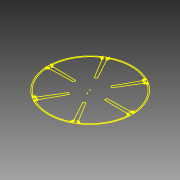
# Autodesk Inventor part: Wheel-190D-Join
Saved by Autodesk Inventor 2014 SP1 (Build 180222100, 222)
## iProperties
Created: 2017-01-25
Part Number: Wheel-190D-Join
Material: Generic
Document SubType Name: Modeling
Designer: danielsikar
Density: 1 g/cm^3
Appearance: Default
Author: danielsikar
Autodesk Inventor part; units mm, degrees
ref_plane "YZ Plane" through (0, 0, 0) normal (1, 0, 0) x (0, 1, 0)
ref_plane "XZ Plane" through (0, 0, 0) normal (0, 1, 0) x (-1, 0, 0)
ref_plane "XY Plane" through (0, 0, 0) normal (0, 0, 1) x (1, 0, 0)
sketch "Sketch1" plane through (0, 0, 0) normal (0, 0, 1) x (1, 0, 0)
  arc A0 (31.6369, 7.0811) -> (31.6369, 12.2394) centre (-3.2679, 9.6603) ccw
  line L0 (31.6369, 12.2394) -> (85.6305, 13.4951)
  spline S0 degree 3 poles (88.553, 15.6009) (88.5581, 15.5214) (88.5526, 15.4427) (88.5217, 15.2843) (88.4962, 15.2066) (88.3926, 14.9703) (88.2868, 14.8191) (87.9731, 14.4565) (87.7042, 14.2313) (87.1267, 13.8761) (86.8348, 13.7414) (86.2409, 13.5562) (85.9366, 13.5022) (85.6305, 13.4951) knots 0 0 0 0 0.068577 0.068577 0.138951 0.138951 0.290932 0.290932 0.552904 0.552904 0.779743 0.779743 1 1 1 1
  arc A1 (88.553, 15.6009) -> (47.7872, 86.2092) centre (-3.2679, 9.6603) ccw
  spline S1 degree 3 poles (44.5024, 84.7311) (44.7113, 85.0744) (44.9886, 85.3747) (45.7206, 85.9508) (46.1829, 86.1728) (46.7972, 86.3435) (47.0239, 86.382) (47.3383, 86.3694) (47.4368, 86.3554) (47.6229, 86.3008) (47.7082, 86.2619) (47.7872, 86.2092) knots 0 0 0 0 0.278386 0.278386 0.644497 0.644497 0.831809 0.831809 0.917649 0.917649 1 1 1 1
  line L1 (16.4181, 38.5991) -> (44.5024, 84.7311)
  arc A2 (16.4181, 38.5991) -> (11.9508, 41.1783) centre (-3.2679, 9.6603) ccw
  line L2 (11.9508, 41.1783) -> (37.8602, 88.566)
  spline S2 degree 3 poles (37.4978, 92.1498) (37.6052, 92.0967) (37.6979, 92.0243) (37.8803, 91.8249) (37.9599, 91.6922) (38.1263, 91.328) (38.198, 91.0566) (38.2844, 90.4211) (38.2862, 90.026) (38.157, 89.2543) (38.0394, 88.8938) (37.8602, 88.566) knots 0 0 0 0 0.107871 0.107871 0.243625 0.243625 0.469812 0.469812 0.746518 0.746518 1 1 1 1
  arc A3 (37.4978, 92.1498) -> (-44.0337, 92.1498) centre (-3.2679, 9.6603) ccw
  spline S3 degree 3 poles (-44.3961, 88.566) (-44.5889, 88.9186) (-44.7103, 89.3089) (-44.8432, 90.2308) (-44.8043, 90.7422) (-44.645, 91.3596) (-44.565, 91.5752) (-44.3969, 91.8411) (-44.3355, 91.9195) (-44.1951, 92.0533) (-44.1189, 92.1077) (-44.0337, 92.1498) knots 0 0 0 0 0.278386 0.278386 0.644497 0.644497 0.831809 0.831809 0.917649 0.917649 1 1 1 1
  line L3 (-18.4867, 41.1783) -> (-44.3961, 88.566)
  arc A4 (-18.4867, 41.1783) -> (-22.954, 38.5991) centre (-3.2679, 9.6603) ccw
  line L4 (-22.954, 38.5991) -> (-51.0383, 84.7311)
  spline S4 degree 3 poles (-54.3231, 86.2092) (-54.2235, 86.2757) (-54.1144, 86.3197) (-53.8505, 86.3781) (-53.6958, 86.3806) (-53.2972, 86.3426) (-53.0263, 86.269) (-52.4327, 86.0261) (-52.0897, 85.8301) (-51.4859, 85.3323) (-51.2325, 85.0503) (-51.0383, 84.7311) knots 0 0 0 0 0.107871 0.107871 0.243625 0.243625 0.469812 0.469812 0.746518 0.746518 1 1 1 1
  arc A5 (-54.3231, 86.2092) -> (-95.0889, 15.6009) centre (-3.2679, 9.6603) ccw
  spline S5 degree 3 poles (-92.1664, 13.4951) (-92.5681, 13.5044) (-92.9668, 13.5944) (-93.8317, 13.9403) (-94.2552, 14.2297) (-94.7102, 14.6763) (-94.8569, 14.8534) (-95.0031, 15.132) (-95.0403, 15.2243) (-95.086, 15.4128) (-95.095, 15.5061) (-95.0889, 15.6009) knots 0 0 0 0 0.278386 0.278386 0.644497 0.644497 0.831809 0.831809 0.917649 0.917649 1 1 1 1
  line L5 (-38.1728, 12.2394) -> (-92.1664, 13.4951)
  arc A6 (-38.1728, 12.2394) -> (-38.1728, 7.0811) centre (-3.2679, 9.6603) ccw
  line L6 (-38.1728, 7.0811) -> (-92.1664, 5.8254)
  spline S6 degree 3 poles (-95.0889, 3.7196) (-95.0966, 3.8392) (-95.0802, 3.9557) (-94.9988, 4.2134) (-94.9236, 4.3486) (-94.6914, 4.6748) (-94.4922, 4.8726) (-93.9851, 5.2652) (-93.6438, 5.4643) (-92.9108, 5.7383) (-92.5399, 5.8167) (-92.1664, 5.8254) knots 0 0 0 0 0.107871 0.107871 0.243625 0.243625 0.469812 0.469812 0.746518 0.746518 1 1 1 1
  arc A7 (-95.0889, 3.7196) -> (-54.3231, -66.8887) centre (-3.2679, 9.6603) ccw
  spline S7 degree 3 poles (-51.0383, -65.4106) (-51.2472, -65.7539) (-51.5245, -66.0542) (-52.2565, -66.6303) (-52.7188, -66.8523) (-53.3331, -67.023) (-53.5598, -67.0615) (-53.8742, -67.0489) (-53.9727, -67.0349) (-54.1588, -66.9803) (-54.2441, -66.9414) (-54.3231, -66.8887) knots 0 0 0 0 0.278386 0.278386 0.644497 0.644497 0.831809 0.831809 0.917649 0.917649 1 1 1 1
  line L7 (-22.954, -19.2786) -> (-51.0383, -65.4106)
  arc A8 (-22.954, -19.2786) -> (-18.4867, -21.8578) centre (-3.2679, 9.6603) ccw
  line L8 (-18.4867, -21.8578) -> (-44.3961, -69.2455)
  spline S8 degree 3 poles (-44.0337, -72.8293) (-44.1411, -72.7762) (-44.2338, -72.7038) (-44.4162, -72.5044) (-44.4958, -72.3717) (-44.6622, -72.0075) (-44.7339, -71.7361) (-44.8203, -71.1006) (-44.8221, -70.7055) (-44.6929, -69.9338) (-44.5753, -69.5733) (-44.3961, -69.2455) knots 0 0 0 0 0.107871 0.107871 0.243625 0.243625 0.469812 0.469812 0.746518 0.746518 1 1 1 1
  arc A9 (-44.0337, -72.8293) -> (37.4978, -72.8293) centre (-3.2679, 9.6603) ccw
  spline S9 degree 3 poles (37.8602, -69.2455) (38.053, -69.598) (38.1744, -69.9884) (38.3073, -70.9103) (38.2684, -71.4217) (38.1091, -72.0391) (38.0291, -72.2547) (37.861, -72.5206) (37.7996, -72.599) (37.6592, -72.7328) (37.583, -72.7872) (37.4978, -72.8293) knots 0 0 0 0 0.278386 0.278386 0.644497 0.644497 0.831809 0.831809 0.917649 0.917649 1 1 1 1
  line L9 (11.9508, -21.8578) -> (37.8602, -69.2455)
  arc A10 (11.9508, -21.8578) -> (16.4181, -19.2786) centre (-3.2679, 9.6603) ccw
  line L10 (16.4181, -19.2786) -> (44.5024, -65.4106)
  spline S10 degree 3 poles (47.7872, -66.8887) (47.6876, -66.9552) (47.5785, -66.9992) (47.3146, -67.0575) (47.1599, -67.0601) (46.7613, -67.0221) (46.4904, -66.9484) (45.8968, -66.7056) (45.5538, -66.5096) (44.95, -66.0118) (44.6966, -65.7298) (44.5024, -65.4106) knots 0 0 0 0 0.107871 0.107871 0.243625 0.243625 0.469812 0.469812 0.746518 0.746518 1 1 1 1
  arc A11 (47.7872, -66.8887) -> (88.553, 3.7196) centre (-3.2679, 9.6603) ccw
  spline S11 degree 3 poles (85.6305, 5.8254) (86.0322, 5.8161) (86.4309, 5.7261) (87.2958, 5.3802) (87.7193, 5.0908) (88.1743, 4.6442) (88.321, 4.4671) (88.4672, 4.1885) (88.5044, 4.0962) (88.5501, 3.9077) (88.5591, 3.8144) (88.553, 3.7196) knots 0 0 0 0 0.278386 0.278386 0.644497 0.644497 0.831809 0.831809 0.917649 0.917649 1 1 1 1
  line L11 (31.6369, 7.0811) -> (85.6305, 5.8254)
  line L12 (90.9918, 13.6198) -> (91.074, 10.0868)
  arc A12 (47.291, -69.9913) -> (91.074, 10.0868) centre (-3.2679, 9.6603) ccw
  line L13 (47.291, -69.9913) -> (40.5213, -74.1126)
  line L14 (40.4329, -73.9508) -> (40.5213, -74.1126)
  arc A13 (-46.9688, -73.9508) -> (40.4329, -73.9508) centre (-3.2679, 9.6603) ccw
  line L15 (-46.9688, -73.9508) -> (-53.9227, -70.1487)
  line L16 (-53.8269, -69.9913) -> (-53.9227, -70.1487)
  arc A14 (-97.5277, 5.7007) -> (-53.8269, -69.9913) centre (-3.2679, 9.6603) ccw
  line L17 (-97.5277, 5.7007) -> (-97.712, 13.6241)
  line L18 (-97.5277, 13.6198) -> (-97.712, 13.6241)
  arc A15 (-53.8269, 89.3118) -> (-97.5277, 13.6198) centre (-3.2679, 9.6603) ccw
  line L19 (-53.8269, 89.3118) -> (-47.0572, 93.4331)
  line L20 (-46.9688, 93.2714) -> (-47.0572, 93.4331)
  arc A16 (40.4329, 93.2714) -> (-46.9688, 93.2714) centre (-3.2679, 9.6603) ccw
  line L21 (40.4329, 93.2714) -> (47.3868, 89.4693)
  line L22 (47.291, 89.3118) -> (47.3868, 89.4693)
  arc A17 (90.9918, 13.6198) -> (47.291, 89.3118) centre (-3.2679, 9.6603) ccw
  point P0 (0, 0)
ref_plane "Work Plane1" through (6.7321, 7.6603, 6.5) normal (0, 0, -1) x (-1, 0, 0)
ref_plane "Work Plane2" through (-91.9966, 5.6978, 0) normal (0, 0, 1) x (1, 0, 0)
sketch "Sketch2" plane through (6.7321, 7.6603, 6.5) normal (0, 0, -1) x (-1, 0, 0)
  arc A0 (-24.9048, 4.5792) -> (-24.9048, -0.5792) centre (10, 2) ccw
  line L0 (-24.9048, 4.5792) -> (-78.8985, 5.8348)
  spline S0 degree 3 poles (-81.8209, 7.9406) (-81.8261, 7.8611) (-81.8206, 7.7825) (-81.7897, 7.6241) (-81.7641, 7.5464) (-81.6606, 7.31) (-81.5548, 7.1589) (-81.2411, 6.7962) (-80.9721, 6.571) (-80.3946, 6.2158) (-80.1028, 6.0812) (-79.5089, 5.8959) (-79.2045, 5.842) (-78.8985, 5.8348) knots 0 0 0 0 0.068577 0.068577 0.138951 0.138951 0.290932 0.290932 0.552904 0.552904 0.779743 0.779743 1 1 1 1
  arc A1 (-41.0552, 78.5489) -> (-81.8209, 7.9406) centre (10, 2) ccw
  spline S1 degree 3 poles (-37.7703, 77.0709) (-37.9792, 77.4141) (-38.2566, 77.7144) (-38.9885, 78.2905) (-39.4509, 78.5125) (-40.0652, 78.6833) (-40.2919, 78.7218) (-40.6062, 78.7092) (-40.7048, 78.6952) (-40.8909, 78.6405) (-40.9762, 78.6017) (-41.0552, 78.5489) knots 0 0 0 0 0.278386 0.278386 0.644497 0.644497 0.831809 0.831809 0.917649 0.917649 1 1 1 1
  line L1 (-9.6861, 30.9389) -> (-37.7703, 77.0709)
  arc A2 (-5.2188, 33.5181) -> (-9.6861, 30.9389) centre (10, 2) ccw
  line L2 (-5.2188, 33.5181) -> (-31.1282, 80.9057)
  spline S2 degree 3 poles (-30.7657, 84.4896) (-30.8731, 84.4365) (-30.9658, 84.364) (-31.1483, 84.1647) (-31.2278, 84.0319) (-31.3942, 83.6678) (-31.4659, 83.3963) (-31.5524, 82.7609) (-31.5541, 82.3658) (-31.4249, 81.594) (-31.3074, 81.2336) (-31.1282, 80.9057) knots 0 0 0 0 0.107871 0.107871 0.243625 0.243625 0.469812 0.469812 0.746518 0.746518 1 1 1 1
  arc A3 (50.7657, 84.4896) -> (-30.7657, 84.4896) centre (10, 2) ccw
  spline S3 degree 3 poles (51.1282, 80.9057) (51.3209, 81.2583) (51.4423, 81.6486) (51.5753, 82.5706) (51.5364, 83.082) (51.3771, 83.6993) (51.2971, 83.9149) (51.129, 84.1809) (51.0676, 84.2592) (50.9272, 84.393) (50.8509, 84.4475) (50.7657, 84.4896) knots 0 0 0 0 0.278386 0.278386 0.644497 0.644497 0.831809 0.831809 0.917649 0.917649 1 1 1 1
  line L3 (25.2188, 33.5181) -> (51.1282, 80.9057)
  arc A4 (29.6861, 30.9389) -> (25.2188, 33.5181) centre (10, 2) ccw
  line L4 (29.6861, 30.9389) -> (57.7703, 77.0709)
  spline S4 degree 3 poles (61.0552, 78.5489) (60.9555, 78.6154) (60.8464, 78.6595) (60.5826, 78.7178) (60.4278, 78.7203) (60.0293, 78.6823) (59.7583, 78.6087) (59.1648, 78.3659) (58.8217, 78.1698) (58.218, 77.672) (57.9646, 77.39) (57.7703, 77.0709) knots 0 0 0 0 0.107871 0.107871 0.243625 0.243625 0.469812 0.469812 0.746518 0.746518 1 1 1 1
  arc A5 (101.8209, 7.9406) -> (61.0552, 78.5489) centre (10, 2) ccw
  spline S5 degree 3 poles (98.8985, 5.8348) (99.3002, 5.8442) (99.6989, 5.9342) (100.5638, 6.28) (100.9872, 6.5694) (101.4422, 7.0161) (101.5889, 7.1931) (101.7352, 7.4717) (101.7724, 7.564) (101.8181, 7.7525) (101.8271, 7.8458) (101.8209, 7.9406) knots 0 0 0 0 0.278386 0.278386 0.644497 0.644497 0.831809 0.831809 0.917649 0.917649 1 1 1 1
  line L5 (44.9048, 4.5792) -> (98.8985, 5.8348)
  arc A6 (44.9048, -0.5792) -> (44.9048, 4.5792) centre (10, 2) ccw
  line L6 (44.9048, -0.5792) -> (98.8985, -1.8348)
  spline S6 degree 3 poles (101.8209, -3.9406) (101.8287, -3.8211) (101.8123, -3.7046) (101.7308, -3.4469) (101.6557, -3.3116) (101.4235, -2.9855) (101.2242, -2.7876) (100.7172, -2.395) (100.3759, -2.196) (99.6429, -1.922) (99.272, -1.8435) (98.8985, -1.8348) knots 0 0 0 0 0.107871 0.107871 0.243625 0.243625 0.469812 0.469812 0.746518 0.746518 1 1 1 1
  arc A7 (61.0552, -74.5489) -> (101.8209, -3.9406) centre (10, 2) ccw
  spline S7 degree 3 poles (57.7703, -73.0709) (57.9792, -73.4141) (58.2566, -73.7144) (58.9885, -74.2905) (59.4509, -74.5125) (60.0652, -74.6833) (60.2919, -74.7218) (60.6062, -74.7092) (60.7048, -74.6952) (60.8909, -74.6405) (60.9762, -74.6017) (61.0552, -74.5489) knots 0 0 0 0 0.278386 0.278386 0.644497 0.644497 0.831809 0.831809 0.917649 0.917649 1 1 1 1
  line L7 (29.6861, -26.9389) -> (57.7703, -73.0709)
  arc A8 (25.2188, -29.5181) -> (29.6861, -26.9389) centre (10, 2) ccw
  line L8 (25.2188, -29.5181) -> (51.1282, -76.9057)
  spline S8 degree 3 poles (50.7657, -80.4896) (50.8731, -80.4365) (50.9658, -80.364) (51.1483, -80.1647) (51.2278, -80.0319) (51.3942, -79.6678) (51.4659, -79.3963) (51.5524, -78.7609) (51.5541, -78.3658) (51.4249, -77.594) (51.3074, -77.2336) (51.1282, -76.9057) knots 0 0 0 0 0.107871 0.107871 0.243625 0.243625 0.469812 0.469812 0.746518 0.746518 1 1 1 1
  arc A9 (-30.7657, -80.4896) -> (50.7657, -80.4896) centre (10, 2) ccw
  spline S9 degree 3 poles (-31.1282, -76.9057) (-31.3209, -77.2583) (-31.4423, -77.6486) (-31.5753, -78.5706) (-31.5364, -79.082) (-31.3771, -79.6993) (-31.2971, -79.9149) (-31.129, -80.1809) (-31.0676, -80.2592) (-30.9272, -80.393) (-30.8509, -80.4475) (-30.7657, -80.4896) knots 0 0 0 0 0.278386 0.278386 0.644497 0.644497 0.831809 0.831809 0.917649 0.917649 1 1 1 1
  line L9 (-5.2188, -29.5181) -> (-31.1282, -76.9057)
  arc A10 (-9.6861, -26.9389) -> (-5.2188, -29.5181) centre (10, 2) ccw
  line L10 (-9.6861, -26.9389) -> (-37.7703, -73.0709)
  spline S10 degree 3 poles (-41.0552, -74.5489) (-40.9555, -74.6154) (-40.8464, -74.6595) (-40.5826, -74.7178) (-40.4278, -74.7203) (-40.0293, -74.6823) (-39.7583, -74.6087) (-39.1648, -74.3659) (-38.8217, -74.1698) (-38.218, -73.672) (-37.9646, -73.39) (-37.7703, -73.0709) knots 0 0 0 0 0.107871 0.107871 0.243625 0.243625 0.469812 0.469812 0.746518 0.746518 1 1 1 1
  arc A11 (-81.8209, -3.9406) -> (-41.0552, -74.5489) centre (10, 2) ccw
  spline S11 degree 3 poles (-78.8985, -1.8348) (-79.3002, -1.8442) (-79.6989, -1.9342) (-80.5638, -2.28) (-80.9872, -2.5694) (-81.4422, -3.0161) (-81.5889, -3.1931) (-81.7352, -3.4717) (-81.7724, -3.564) (-81.8181, -3.7525) (-81.8271, -3.8458) (-81.8209, -3.9406) knots 0 0 0 0 0.278386 0.278386 0.644497 0.644497 0.831809 0.831809 0.917649 0.917649 1 1 1 1
  line L11 (-24.9048, -0.5792) -> (-78.8985, -1.8348)
  line L12 (-84.2597, 5.9595) -> (-84.3419, 2.4266)
  arc A12 (-84.3419, 2.4266) -> (-40.5589, -77.6516) centre (10, 2) ccw
  line L13 (-40.5589, -77.6516) -> (-33.7892, -81.7728)
  line L14 (-33.7008, -81.6111) -> (-33.7892, -81.7728)
  arc A13 (-33.7008, -81.6111) -> (53.7008, -81.6111) centre (10, 2) ccw
  line L15 (53.7008, -81.6111) -> (60.6548, -77.809)
  line L16 (60.5589, -77.6516) -> (60.6548, -77.809)
  arc A14 (60.5589, -77.6516) -> (104.2597, -1.9595) centre (10, 2) ccw
  line L17 (104.2597, -1.9595) -> (104.444, 5.9638)
  line L18 (104.2597, 5.9595) -> (104.444, 5.9638)
  arc A15 (104.2597, 5.9595) -> (60.5589, 81.6516) centre (10, 2) ccw
  line L19 (60.5589, 81.6516) -> (53.7892, 85.7728)
  line L20 (53.7008, 85.6111) -> (53.7892, 85.7728)
  arc A16 (53.7008, 85.6111) -> (-33.7008, 85.6111) centre (10, 2) ccw
  line L21 (-33.7008, 85.6111) -> (-40.6548, 81.809)
  line L22 (-40.5589, 81.6516) -> (-40.6548, 81.809)
  arc A17 (-40.5589, 81.6516) -> (-84.2597, 5.9595) centre (10, 2) ccw
  point P0 (6.7321, -7.6603)
extrude "Extrusion1" add sketch "Sketch2" along normal up to surface (6.5 mm away)
ref_plane "Work Plane3" through (-3.2679, 9.6603, 1.5) normal (0, 0, 1) x (1, 0, 0)
sketch "Sketch3" plane through (-3.2679, 9.6603, 1.5) normal (0, 0, 1) x (1, 0, 0)
  circle A0 centre (0, 0) radius 35
  circle A1 centre (0, 0) radius 37.5
  point P0 (3.2679, -9.6603)
  dimension "d2" = 70
  dimension "d3" = 75
  constraints: 2 centre point, 1 coincident
  measures "d2" diameter of A0
  measures "d3" diameter of A1
ref_plane "Work Plane4" through (11.9508, 38.5991, 10.5) normal (0, 0, 1) x (1, 0, 0)
extrude "Extrusion2" add sketch "Sketch3" along normal up to surface (9 mm away)
sketch "Sketch4" plane through (-3.2679, 9.6603, 1.5) normal (0, 0, -1) x (-1, 0, 0)
  arc A0 (-16.4195, -33.7142) -> (16.4195, -33.7142) centre (0, 0) ccw projected
  circle A1 centre (0, 0) radius 35
  circle A2 centre (0, 0) radius 37.5
  point P0 (-3.2679, -9.6603)
  dimension "d6" = 70
  dimension "d7" = 75
  constraints: 2 centre point, 2 coincident
  measures "d6" diameter of A1
  measures "d7" diameter of A2
extrude "Extrusion3" add sketch "Sketch4" along normal up to surface (1.5 mm away)
body "Solid1"
